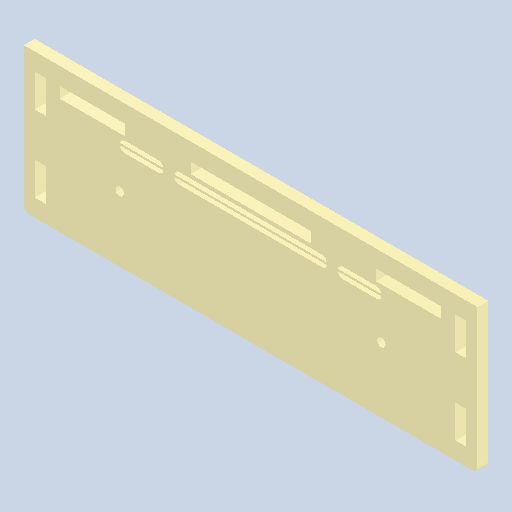
# Autodesk Inventor part: case bottom front
Saved by Autodesk Inventor 2022 (Build 260153000, 153)
## iProperties
Created: 2021-05-28
Part Number: case bottom front
Material: Nylon, molybdenum disulphide
Document SubType Name: Modeling
Designer: benka
Density: 1.13 g/cm^3
Appearance: Nylon 6
Author: benka
Autodesk Inventor part; units mm, degrees
ref_plane "YZ Plane" through (0, 0, 0) normal (1, 0, 0) x (0, 1, 0)
ref_plane "XZ Plane" through (0, 0, 0) normal (0, 1, 0) x (-1, 0, 0)
ref_plane "XY Plane" through (0, 0, 0) normal (0, 0, 1) x (1, 0, 0)
sketch "Sketch1" plane through (0, 0, 0) normal (0, 0, 1) x (1, 0, 0)
  line L0 (-101.9973, -32.9991) -> (101.9973, -32.9991)
  line L1 (-101.9973, 33.0009) -> (101.9973, 33.0009)
  line L2 (-103.9973, -30.9991) -> (-103.9973, 31.0009)
  line L3 (103.9973, 31.0009) -> (103.9973, -30.9991)
  arc A0 (-103.9973, -30.9991) -> (-101.9973, -32.9991) centre (-101.9973, -30.9991) ccw
  arc A1 (101.9973, -32.9991) -> (103.9973, -30.9991) centre (101.9973, -30.9991) ccw
  line L4 (103.9973, 31.0009) -> (103.9973, 33.0009)
  line L5 (101.9973, 33.0009) -> (103.9973, 33.0009)
  line L6 (-103.9973, 31.0009) -> (-103.9973, 33.0009)
  line L7 (-101.9973, 33.0009) -> (-103.9973, 33.0009)
  line L8 (57.998, 18.2189) -> (41.998, 18.2189)
  line L9 (41.998, 13.2189) -> (57.998, 13.2189)
  line L10 (-58.002, 18.2189) -> (-42.002, 18.2189)
  line L11 (-42.002, 13.2189) -> (-58.002, 13.2189)
  line L12 (32.998, 18.2189) -> (-33.002, 18.2189)
  line L13 (-33.002, 13.2189) -> (32.998, 13.2189)
  arc A2 (34.998, 16.2189) -> (32.998, 18.2189) centre (32.998, 16.2189) ccw
  arc A3 (-35.002, 15.2189) -> (-33.002, 13.2189) centre (-33.002, 15.2189) ccw
  arc A4 (-33.002, 18.2189) -> (-35.002, 16.2189) centre (-33.002, 16.2189) ccw
  arc A5 (-40.002, 16.2189) -> (-42.002, 18.2189) centre (-42.002, 16.2189) ccw
  arc A6 (-42.002, 13.2189) -> (-40.002, 15.2189) centre (-42.002, 15.2189) ccw
  arc A7 (-60.002, 15.2189) -> (-58.002, 13.2189) centre (-58.002, 15.2189) ccw
  arc A8 (-58.002, 18.2189) -> (-60.002, 16.2189) centre (-58.002, 16.2189) ccw
  arc A9 (39.998, 15.2189) -> (41.998, 13.2189) centre (41.998, 15.2189) ccw
  arc A10 (41.998, 18.2189) -> (39.998, 16.2189) centre (41.998, 16.2189) ccw
  arc A11 (59.998, 16.2189) -> (57.998, 18.2189) centre (57.998, 16.2189) ccw
  arc A12 (57.998, 13.2189) -> (59.998, 15.2189) centre (57.998, 15.2189) ccw
  arc A13 (32.998, 13.2189) -> (34.998, 15.2189) centre (32.998, 15.2189) ccw
  line L14 (59.998, 16.2189) -> (39.998, 16.2189)
  line L15 (39.998, 15.2189) -> (59.998, 15.2189)
  line L16 (34.998, 16.2189) -> (-35.002, 16.2189)
  line L17 (-35.002, 15.2189) -> (34.998, 15.2189)
  line L18 (-40.002, 16.2189) -> (-60.002, 16.2189)
  line L19 (-60.002, 15.2189) -> (-40.002, 15.2189)
  circle A14 centre (-59.9992, -3) radius 2
  circle A15 centre (59.9979, -3) radius 2
  line L20 (93.998, -24.9998) -> (93.998, -10.0006)
  line L21 (93.998, -10.0006) -> (98.998, -10.0006)
  line L22 (98.998, -24.9998) -> (98.998, -10.0006)
  line L23 (93.998, -24.9998) -> (98.998, -24.9998)
  line L24 (93.998, 9.9994) -> (93.998, 25.0009)
  line L25 (93.998, 25.0009) -> (98.998, 25.0009)
  line L26 (98.998, 9.9994) -> (98.998, 25.0009)
  line L27 (93.998, 9.9994) -> (98.998, 9.9994)
  line L28 (87.498, 20.0009) -> (57.498, 20.0009)
  line L29 (57.498, 20.0009) -> (57.498, 25.0009)
  line L30 (87.498, 25.0009) -> (57.498, 25.0009)
  line L31 (87.498, 20.0009) -> (87.498, 25.0009)
  line L32 (27.498, 20.0009) -> (-27.502, 20.0009)
  line L33 (-27.502, 20.0009) -> (-27.502, 25.0009)
  line L34 (27.498, 25.0009) -> (-27.502, 25.0009)
  line L35 (27.498, 20.0009) -> (27.498, 25.0009)
  line L36 (-57.502, 20.0009) -> (-87.502, 20.0009)
  line L37 (-87.502, 20.0009) -> (-87.502, 25.0009)
  line L38 (-57.502, 25.0009) -> (-87.502, 25.0009)
  line L39 (-57.502, 20.0009) -> (-57.502, 25.0009)
  line L40 (-99.002, 9.9994) -> (-99.002, 25.0009)
  line L41 (-99.002, 25.0009) -> (-94.002, 25.0009)
  line L42 (-94.002, 9.9994) -> (-94.002, 25.0009)
  line L43 (-99.002, 9.9994) -> (-94.002, 9.9994)
  line L44 (-99.002, -24.9998) -> (-99.002, -10.0006)
  line L45 (-99.002, -10.0006) -> (-94.002, -10.0006)
  line L46 (-94.002, -24.9998) -> (-94.002, -10.0006)
  line L47 (-99.002, -24.9998) -> (-94.002, -24.9998)
  point P0 (-85.2166, -15.942)
  point P1 (-103.9973, -32.9991)
  point P2 (103.9973, -32.9991)
  point P3 (59.998, 18.2189)
  point P4 (59.998, 13.2189)
  point P5 (-60.002, 16.2189)
  point P6 (59.998, 15.2189)
  point P7 (59.9979, -3)
extrude "Extrusion1" add sketch "Sketch1" along normal blind 5
body "Solid1"
